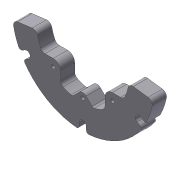
# Autodesk Inventor part: IFI_Wheel_Weight_8in
Saved by Autodesk Inventor 2012 (Build 160160000, 160)
## iProperties
Created: 2012-01-22
Part Number: IFI_Wheel_Weight_8in
Material: Aluminum-6061
Document SubType Name: Modeling
Designer: JesseK
Mass: 396.965 g
Surface Area: 273.467 cm^2
Volume: 146.481 cm^3
Density: 2.71 g/cm^3
Author: JesseK
Autodesk Inventor part; units mm, degrees
ref_plane "YZ Plane" through (0, 0, 0) normal (1, 0, 0) x (0, 1, 0)
ref_plane "XZ Plane" through (0, 0, 0) normal (0, 1, 0) x (-1, 0, 0)
ref_plane "XY Plane" through (0, 0, 0) normal (0, 0, 1) x (1, 0, 0)
sketch "Sketch1" plane through (0, 0, 0) normal (0, 0, 1) x (1, 0, 0)
  line L0 (0, 0) -> (-61.1827, -8.0012) construction
  line L1 (61.2899, -8.1227) -> (0, 0) construction
  line L2 (86.7988, -11.5034) -> (67.2983, -8.919)
  line L3 (-67.1847, -8.7862) -> (-86.5468, -11.3183)
  line L4 (0, 0) -> (0, -62.0753) construction
  line L5 (61.2899, -8.1227) -> (0, -62.0753) construction
  line L6 (-61.1827, -8.0012) -> (0, -62.0753) construction
  arc A0 (-29.7125, -39.3071) -> (-39.2375, -29.7799) centre (-39.2375, -39.3049) ccw
  arc A1 (-60.1692, -13.6752) -> (-55.9036, -26.1177) centre (0, 0) ccw
  arc A2 (56.0545, -26.1271) -> (60.2727, -13.8035) centre (0.1394, -0.1047) ccw
  line L7 (-50.1505, -29.7799) -> (-39.2375, -29.7799)
  line L8 (-29.7125, -39.3071) -> (-29.7151, -50.2201)
  arc A3 (39.3667, -29.7672) -> (29.6251, -39.4816) centre (39.3395, -39.4816) ccw
  line L9 (29.6251, -39.4816) -> (29.6251, -50.3946)
  line L10 (39.3667, -29.7672) -> (50.2797, -29.7978)
  circle A4 centre (0.1394, -0.1047) radius 55.5625 construction
  line L11 (-39.2375, -39.3049) -> (0.1394, -0.1047) construction
  line L12 (0.1394, -0.1047) -> (39.3395, -39.4816) construction
  line L13 (39.3395, -39.4816) -> (0, -62.0753) construction
  line L14 (-39.2375, -39.3049) -> (0, -62.0753) construction
  circle A5 centre (-39.2375, -39.3049) radius 2.4384
  circle A6 centre (39.3395, -39.4816) radius 2.4384
  arc A7 (-91.9453, -18.8835) -> (-85.1324, -39.6138) centre (0.1394, -0.1047) ccw
  arc A8 (-76.9964, -53.7918) -> (-8.2199, -93.7122) centre (0.1394, -0.1047) ccw
  arc A9 (8.2102, -93.7375) -> (77.1094, -54.0293) centre (0.1394, -0.1047) ccw
  arc A10 (83.8051, -42.9099) -> (92.1837, -19.0805) centre (0.1394, -0.1047) ccw
  line L15 (-93.0629, -12.1704) -> (-83.6165, -42.7332) construction
  line L16 (-78.9151, -50.9242) -> (-4.7625, -93.9568) construction
  line L17 (4.7625, -93.9709) -> (79.0426, -51.1588) construction
  line L18 (83.8051, -42.9099) -> (93.316, -12.3671) construction
  line L19 (0, -62.0753) -> (0, -103.9027) construction
  line L20 (-4.7625, -90.5498) -> (-4.7625, -86.0193)
  line L21 (4.7625, -86.0193) -> (4.7625, -90.5743)
  arc A11 (4.7625, -86.0193) -> (-4.7625, -86.0193) centre (0, -86.0193) ccw
  line L22 (0.1394, -0.1047) -> (81.6013, -47.1368) construction
  line L23 (83.8051, -42.9099) -> (76.9144, -38.9315)
  line L24 (72.1519, -47.1804) -> (76.0966, -49.4579)
  arc A12 (76.9144, -38.9315) -> (72.1519, -47.1804) centre (74.5331, -43.0559) ccw
  line L25 (0.1394, -0.1047) -> (-92.6905, -53.7001) construction
  line L26 (-80.6641, -41.0286) -> (-76.7766, -38.7842)
  line L27 (-72.0545, -46.9632) -> (-75.978, -49.2284)
  arc A13 (-72.0545, -46.9632) -> (-76.7766, -38.7842) centre (-74.4155, -42.8737) ccw
  arc A14 (-86.5468, -11.3183) -> (-91.9453, -18.8835) centre (-85.7234, -17.6146) ccw
  arc A15 (-60.1692, -13.6752) -> (-67.1847, -8.7862) centre (-66.3613, -15.0825) ccw
  arc A16 (-55.9036, -26.1177) -> (-50.1505, -29.7799) centre (-50.1505, -23.4299) ccw
  arc A17 (-29.7151, -50.2201) -> (-25.945, -56.0239) centre (-23.3651, -50.2216) ccw
  arc A18 (25.7485, -56.2431) -> (29.6251, -50.3946) centre (23.2751, -50.3946) ccw
  arc A19 (50.2797, -29.7978) -> (56.0545, -26.1271) centre (50.2975, -23.4478) ccw
  arc A20 (67.2983, -8.919) -> (60.2727, -13.8035) centre (66.464, -15.2139) ccw
  arc A21 (92.1837, -19.0805) -> (86.7988, -11.5034) centre (85.9645, -17.7983) ccw
  arc A22 (-85.1324, -39.6138) -> (-80.6641, -41.0286) centre (-82.2516, -38.279) ccw
  arc A23 (-75.978, -49.2284) -> (-76.9964, -53.7918) centre (-74.3905, -51.9781) ccw
  arc A24 (-8.2199, -93.7122) -> (-4.7625, -90.5498) centre (-7.9375, -90.5498) ccw
  arc A25 (4.7625, -90.5743) -> (8.2102, -93.7375) centre (7.9375, -90.5743) ccw
  arc A26 (77.1094, -54.0293) -> (76.0966, -49.4579) centre (74.5091, -52.2075) ccw
  arc A27 (4.5025, -51.1894) -> (-4.48, -51.1668) centre (0, -55.667) ccw
  arc A28 (-25.945, -56.0239) -> (-15.3876, -59.8229) centre (0.1394, -0.1047) ccw
  arc A29 (15.3666, -59.9) -> (25.7485, -56.2431) centre (0.1394, -0.1047) ccw
  line L28 (-4.48, -51.1668) -> (-12.3487, -59.0002)
  line L29 (4.5025, -51.1894) -> (12.3318, -59.0621)
  arc A30 (-15.3876, -59.8229) -> (-12.3487, -59.0002) centre (-14.5887, -56.75) ccw
  arc A31 (12.3318, -59.0621) -> (15.3666, -59.9) centre (14.5831, -56.8232) ccw
  circle A32 centre (0, -55.667) radius 2.4384
  point P0 (-54.0417, -29.7799)
  point P1 (-29.716, -54.3478)
  point P2 (29.6251, -54.3566)
  point P3 (54.1888, -29.8087)
  point P4 (-13.611, -60.2568)
  point P5 (13.5878, -60.325)
  dimension "d2" = 165
  dimension "d5" = 9.525
  dimension "d7" = 111.125
  dimension "d8" = 4.8768
  dimension "d9" = 93.98
  dimension "d10" = 4.7625
  dimension "d11" = 60
  dimension "d12" = 7.9375
  dimension "d13" = 60
  dimension "d16" = 6.35
  dimension "d17" = 3.175
  dimension "d18" = 6.35
  dimension "d19" = 3.175
  constraints: 74 point on circle, 61 end point, 40 tangent, 33 centre point, 20 equal radius, 18 point on line, 12 coincident, 10 equal length, 5 parallel, 5 vertical, 2 collinear, 2 perpendicular, 1 horizontal
  measures "d2" angle of L1 L0
  measures "d5" radius of A0
  measures "d7" diameter of A4
  measures "d8" diameter of A6
  measures "d9" radius of A8
  measures "d10" radius of A11
  measures "d11" angle of L22 L19
  measures "d12" distance of L16.end L20.end
  measures "d13" angle of L19 L25
  measures "d16" radius of A14
  measures "d17" radius of A22
  measures "d18" radius of A27
  measures "d19" radius of A30
extrude "Extrusion3" add sketch "Sketch1" along normal blind 19.05
body "Solid3"
